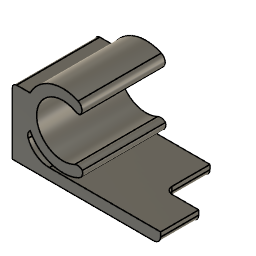
TRUNK BAR SUPPORT (Autodesk Fusion 360 design; units mm, degrees)
Autodesk Fusion 360 part; units mm, degrees
sketch "Sketch1" plane through (0, 0, 0) normal (0, 1, 0) x (1, 0, 0)
  circle A0 centre (0, 0) radius 11.65
  line L0 (7.025, -9.2936) -> (10.2831, -12.5825)
  line L1 (-27, 0) -> (27, 0) construction
  line L2 (7.025, 9.2936) -> (10.2831, 12.5825)
  line L3 (-14.5423, -7.2515) -> (-14.5423, 7.2515)
  arc A1 (-14.5423, -7.2515) -> (-14.5423, 7.2515) centre (0, 0) ccw
  dimension "d1" = 23.3
  constraint coincident A0.centre A1.centre
  constraint coincident A0 L0.start
  constraint coincident L0.end A1
  constraint horizontal L1
  constraint symmetric L0.start L1 L2.start
  constraint symmetric L0.end L1 L2.end
  constraint perpendicular L1 L3
  constraint concentric A0 A1
  measures "d1" diameter of A0
extrude "Extrude1" add sketch "Sketch1" along normal blind 37 contours A0 L0 L2 L3 A1
sketch "Sketch2" plane through (-14.5423, 0, 0) normal (-1, 0, 0) x (0, -1, 0)
  line L0 (0, -7.2515) -> (0, 7.2515)
  line L1 (0, 7.2515) -> (-37, 7.2515)
  line L2 (-37, 7.2515) -> (-37, -7.2515)
  line L3 (-37, -7.2515) -> (0, -7.2515)
  line L4 (-37, 7.2515) -> (0, 7.2515)
  line L5 (0, 7.2515) -> (0, -7.2515)
  line L6 (0, -7.2515) -> (-37, -7.2515)
  line L7 (-37, -7.2515) -> (-37, 7.2515)
  constraint horizontal L4
  constraint vertical L5
  constraint horizontal L6
  constraint vertical L7
  constraint coincident L0.start L3.end
  constraint coincident L1.end L2.start
extrude "Extrude2" add sketch "Sketch2" along normal blind 8
sketch "Sketch3" plane through (0, 0, 0) normal (0, -1, 0) x (1, 0, 0)
  line L0 (10.2831, -12.5825) -> (7.025, -9.2936)
  arc A0 (7.025, 9.2936) -> (7.025, -9.2936) centre (0, 0) ccw
  line L1 (7.025, 9.2936) -> (10.2831, 12.5825)
  arc A1 (10.2831, 12.5825) -> (-14.5423, 7.2515) centre (0, 0) ccw
  line L2 (-14.5423, 7.2515) -> (-22.5423, 7.2515)
  line L3 (-22.5423, 7.2515) -> (-22.5423, -7.2515)
  line L4 (-22.5423, -7.2515) -> (-14.5423, -7.2515)
  arc A2 (-14.5423, -7.2515) -> (10.2831, -12.5825) centre (0, 0) ccw
  line L5 (-22.5423, 0) -> (-22.5423, -50) construction
  line L6 (-11.0827, -22.2515) -> (43.4577, -22.2515)
  line L7 (43.4577, -22.2515) -> (43.4577, -17.2515)
  line L8 (43.4577, -17.2515) -> (-12.9951, -17.2515)
  line L9 (-12.9951, -17.2515) -> (-16.6348, -7.2515)
  line L10 (-22.5423, -7.2515) -> (-22.5423, -22.2515)
  line L11 (-22.5423, -22.2515) -> (-11.0827, -22.2515)
  dimension "d18" = 15
  dimension "d39" = 5
  dimension "d40" = 66
  constraint coincident L3.end L4.start
  constraint midpoint L3 L5.start
  constraint parallel L3 L5
  constraint horizontal L6
  constraint perpendicular L6 L7
  constraint perpendicular L7 L8
  constraint coincident L4 L9.end
  constraint coincident L5 L10.end
  constraint horizontal L11
  measures "d18" vertical distance of L6.start L3.end
  measures "d39" distance of L6.end L7.end
  measures "d40" distance of L7 L10
extrude "Extrude3" add sketch "Sketch3" against normal blind 37
sketch "Sketch6" plane through (0, 0, -17.2515) normal (0, 0, 1) x (-1, 0, 0)
  line L0 (12.9951, 0) -> (-43.4577, 0)
  line L1 (-43.4577, 0) -> (-43.4577, -37)
  line L2 (-43.4577, -37) -> (12.9951, -37)
  line L3 (12.9951, -37) -> (12.9951, 0)
  line L4 (-43.4577, -37) -> (-28.4577, -37)
  line L5 (-28.4577, -37) -> (-28.4577, -17)
  line L6 (-28.4577, -17) -> (-43.4577, -17)
  line L7 (-43.4577, -17) -> (-43.4577, -37)
  dimension "d20" = 20
  dimension "d21" = 15
  constraint horizontal L4
  constraint vertical L5
  constraint horizontal L6
  constraint vertical L7
  constraint coincident L1.end L2.start
  measures "d20" distance of L1.end L6.end
  measures "d21" distance of L5.end L6.end
extrude "Extrude6" cut sketch "Sketch6" against normal blind 20 contours L1 L2 L4 L5 L6 L7
fillet "Fillet1" radius 3 3 edges at (43.4577, 8.5, -22.2515) (28.4577, 27, -22.2515) (28.4577, 17, -19.7515)
fillet "Fillet2" radius 10 1 edges at (-12.9951, 18.5, -17.2515)
fillet "Fillet5" radius 2 1 edges at (-22.5423, 18.5, 7.2515)
fillet "Fillet6" radius 3 4 edges at (10.2831, 18.5, 12.5825) (7.025, 18.5, 9.2936) (7.025, 18.5, -9.2936) (10.2831, 18.5, -12.5825)
fillet "Fillet7" radius 3 1 edges at (-16.6348, 18.5, -7.2515)
equation "d5 = 13 mm - 5 mm"
equation "d40 = 65 mm + 1 mm"
